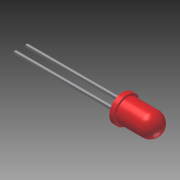
# Autodesk Inventor part: LED 5mm Red height 1-20mm
Saved by Autodesk Inventor 2015 (Build 190159000, 159)
## iProperties
Created: 2011-12-22
Part Number: LED 5mm Red height 1-20mm
Material: Genérico
Document SubType Name: Modeling
Designer: Rod
Density: 1 g/cm^3
Appearance: Valor por defecto
Author: Rod
Autodesk Inventor part; units mm, degrees
ref_plane "YZ Plane" through (0, 0, 0) normal (1, 0, 0) x (0, 1, 0)
ref_plane "XZ Plane" through (0, 0, 0) normal (0, 1, 0) x (-1, 0, 0)
ref_plane "XY Plane" through (0, 0, 0) normal (0, 0, 1) x (1, 0, 0)
sketch "Sketch1" plane through (0, 0, 0) normal (0, 0, 1) x (1, 0, 0)
  line L0 (-33.5517, 0) -> (33.5517, 0)
  line L1 (0, 0) -> (0, 2.95)
  line L2 (0, 2.95) -> (1, 2.95)
  line L3 (1, 2.95) -> (1, 2.5)
  line L4 (1, 2.5) -> (6.1, 2.5)
  arc A0 (8.6, 0) -> (6.1, 2.5) centre (6.1, 0) ccw
  line L5 (8.6, 0) -> (0, 0)
  dimension "d1" = 2.95
  dimension "d2" = 1
  dimension "d3" = 5
  dimension "d4" = 8.6
  dimension "d5" = 2.5
  constraints: 12 end point, 3 point on line, 2 parallel, 2 perpendicular, 2 point on circle, 1 centre point, 1 coincident, 1 collinear, 1 horizontal, 1 midpoint, 1 tangent
  measures "d1" distance of L1.start L1.end
  measures "d2" distance of L1.end L2.end
  measures "d3" diameter of L4.end L0
  measures "d4" distance of L1.start L5.start
  measures "d5" radius of A0
revolve "Revolution1" add sketch "Sketch1" angle 360 about axis through (-33.5517, 0, 0) along (1, 0, 0)
sketch "Sketch2" plane through (0, 0, 0) normal (-1, 0, 0) x (0, 0, 1)
  circle A0 centre (0, 0) radius 2.95 projected
  line L0 (-0.25, 1.52) -> (0.25, 1.52)
  line L1 (0.25, 1.52) -> (0.25, 1.02)
  line L2 (0.25, 1.02) -> (-0.25, 1.02)
  line L3 (-0.25, 1.02) -> (-0.25, 1.52)
  line L4 (-0.25, -1.02) -> (0.25, -1.02)
  line L5 (0.25, -1.02) -> (0.25, -1.52)
  line L6 (0.25, -1.52) -> (-0.25, -1.52)
  line L7 (-0.25, -1.52) -> (-0.25, -1.02)
  line L8 (-0.25, 1.27) -> (0.25, 1.27) construction
  line L9 (-0.25, -1.27) -> (0.25, -1.27) construction
  point P0 (0, 1.52)
  point P1 (0, -1.02)
  dimension "d7" = 0.5
  dimension "d8" = 0.5
  dimension "d9" = 1.27
  dimension "d10" = 1.27
  constraints: 20 end point, 6 midpoint, 4 parallel, 2 equal length, 2 horizontal, 2 perpendicular, 2 vertical alignment
  measures "d7" distance of L0.start L0.end
  measures "d8" distance of L0.end L1.end
  measures "d9" distance from line of A0.centre L8
  measures "d10" distance from line of A0.centre L9
extrude "Extrusion1" add sketch "Sketch2" along normal blind 22.6 contours L0 L1 L2 L3 | L4 L5 L6 L7
sketch "Sketch4" plane through (0, 0, 0) normal (-1, 0, 0) x (0, 0, 1)
  line L0 (-0.25, 1.52) -> (0.25, 1.52) projected
  circle A0 centre (0, 0) radius 2.95 projected
  circle A1 centre (0, 0) radius 2.5 projected
  line L1 (-1.566, 2.5) -> (1.566, 2.5)
  point P0 (0, 2.5)
  constraints: 2 end point, 2 point on circle, 1 midpoint, 1 parallel, 1 vertical alignment, 1 other
extrude "Extrusion2" cut sketch "Sketch4" against normal through all contours L1 A0 picked at (-0.846, 2.5951)
sketch "Sketch3" plane through (-22.6, 0, 0) normal (-1, 0, 0) x (0, 0, 1)
  line L0 (0.25, 1.52) -> (0.25, 1.02) projected
  line L1 (-0.25, 1.52) -> (0.25, 1.52) projected
  line L2 (-0.25, 1.02) -> (-0.25, 1.52) projected
  line L3 (0.25, 1.02) -> (-0.25, 1.02) projected
  line L4 (0.25, -1.02) -> (0.25, -1.52) projected
  line L5 (-0.25, -1.02) -> (0.25, -1.02) projected
  line L6 (-0.25, -1.52) -> (-0.25, -1.02) projected
  line L7 (0.25, -1.52) -> (-0.25, -1.52) projected
  point P0 (0, 0)
  point P1 (0, 1.27)
  point P2 (0, -1.27)
  point P3 (-0.25, 1.27)
  point P4 (-0.25, -1.27)
  constraints: 2 horizontal alignment, 2 midpoint, 2 vertical alignment
equation "\"d10\" = d9"
equation "\"Lead_solder\" = 1"
body "Solid1"
